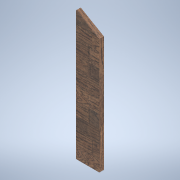
# Autodesk Inventor part: Part1
Saved by Autodesk Inventor 2020 (Build 240168000, 168)
## iProperties
Created: 2020-07-20
Part Number: Part1
Material: Generic
Document SubType Name: Modeling
Designer: Abbas
Density: 1 g/cm^3
Appearance: Default
Author: Abbas
Autodesk Inventor part; units mm, degrees
ref_plane "YZ Plane" through (0, 0, 0) normal (1, 0, 0) x (0, 1, 0)
ref_plane "XZ Plane" through (0, 0, 0) normal (0, 1, 0) x (-1, 0, 0)
ref_plane "XY Plane" through (0, 0, 0) normal (0, 0, 1) x (1, 0, 0)
sketch "Sketch1" plane through (0, 0, 0) normal (0, 0, 1) x (1, 0, 0)
  line L0 (50, 829.4999) -> (50, 329.4999)
  line L1 (50, 329.4999) -> (-50, 329.4999)
  line L2 (-50, 329.4999) -> (-50, 829.4999)
  line L3 (-50, 829.4999) -> (-50, 887.2349)
  line L4 (-50, 829.4999) -> (7.735, 829.4999) construction
  line L5 (-50, 887.2349) -> (50, 829.4999)
  dimension "d2" = 57.735
  dimension "d3" = 90
  dimension "d6" = 500
  dimension "d7" = 500
  constraints: 12 end point, 1 horizontal, 1 parallel, 1 perpendicular, 1 vertical
  measures "d2" distance of L2.end L3.end
  measures "d3" angle of L4 L3
  measures "d6" distance of L0.start L0.end
  measures "d7" distance of L1.end L2.end
extrude "Extrusion1" add sketch "Sketch1" along normal blind 20
body "Solid1"
